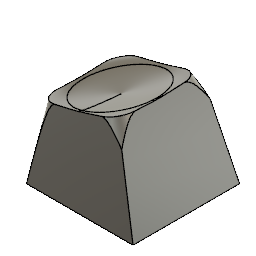
C64 Key Replacement v2 (Autodesk Fusion 360 design; units mm, degrees)
Autodesk Fusion 360 part; units mm, degrees
sketch "Sketch1" plane through (0, 0, 0) normal (0, 1, 0) x (1, 0, 0)
  line L0 (0, 0) -> (18, 0)
  line L1 (18, 0) -> (18, 18)
  line L2 (18, 18) -> (0, 18)
  line L3 (0, 18) -> (0, 0)
  dimension "d1" = 18
  dimension "d2" = 18
  constraint horizontal L0
  constraint vertical L1
  constraint horizontal L2
  constraint vertical L3
  constraint coincident L0.start L3.end
  measures "d1" distance of L0.start L0.end
  measures "d2" distance of L0.start L2.end
extrude "Extrude1" add sketch "Sketch1" along normal blind 15 contours L0 L1 L2 L3 picked at (6, 12)
sketch "Sketch2" plane through (0, 0, 0) normal (0, 0, 1) x (1, 0, 0)
  line L0 (0, 0) -> (0, 11.25)
  line L1 (0, 15) -> (18, 15)
  line L2 (18, 15) -> (0, 15)
  line L3 (0, 11.25) -> (13.507779, 15)
  line L4 (0, 0) -> (0, 6.2)
  spline S0 degree 5 poles (13.507779, 15) (13.660726, 14.651818) (13.961323, 13.959498) (14.396337, 12.933144) (14.944058, 11.589334) (15.571035, 9.953608) (16.134524, 8.366359) (16.628192, 6.832422) (17.046816, 5.355785) (17.390291, 3.936529) (17.663, 2.571306) (17.828559, 1.519298) (17.92492, 0.751524) (17.977, 0.248961) (18, 0) knots 0 0 0 0 0 0 0.1 0.2 0.3 0.4 0.5 0.6 0.7 0.8 0.9 1 1 1 1 1 1
  line L5 (18, 0) -> (0, 0)
  point P0 (16.8, 6.2)
  point P1 (18, 0)
  dimension "d5" = 11.25
  dimension "d7" = 16.8
  constraint coincident L0.start L4.start
  constraint coincident P1 S0.end
  measures "d5" distance of L0.start L0.end
  measures "d7" distance of L4.end P0
extrude "Extrude2" cut sketch "Sketch2" against normal blind 18 contours L0 L3 L4 S0 L5 picked at (9.950869, 9.63052) keep common part
move_body "Move1" bodies 1 to x (-0.96363045, 0.26723838, 0) y (-0.26723838, -0.96363045, 0) z (0, 0, 1) at (14.506577, 23.659133, 0)
move_body "Move2" bodies 1 to x (1, 0, 0) y (0, 1, 0) z (0, 0, 1) at (0, -13, 0)
sketch "Sketch3" plane through (0, 0, 0) normal (1, 0, 0) x (0, 0, -1)
  line L0 (18, -0.181709) -> (0, -0.181709)
  line L1 (9, -0.181709) -> (15.999997, -0.187866)
  line L2 (9, -0.181709) -> (2.000003, -0.18822)
  line L3 (0, 15.469424) -> (18, 15.469424)
  line L4 (0, 15.469424) -> (0, 10.659133)
  line L5 (2.000003, -0.18822) -> (0, 10.659133)
  line L6 (0, 10.659133) -> (0, 15.469424)
  line L7 (15.999997, -0.187866) -> (18, 10.659133)
  line L8 (18, 10.659133) -> (18, 15.469424)
  point P0 (0, 10.659133)
  point P1 (0, 10.659133)
  point P2 (18, 10.659133)
  dimension "d10" = 7
  dimension "d11" = 7
extrude "Extrude3" cut sketch "Sketch3" along normal mid plane 130 contours L0 L3 L4 L5 L6 L7 L8 picked at (9, 7.045519) keep common part
loft "Loft1" cut section 1 face at (6.827078, -0.181709, -11.333689) section 2 face at (8.724795, 12.262564, -12) keep common part
sketch "Sketch4" plane through (0, -0.181709, 0) normal (0, -1, 0) x (1, 0, 0)
  line L0 (11.500146, -16.001132) -> (11.500146, -1.998803)
  line L1 (11.500146, -1.998803) -> (-2.519057, -1.998803)
  line L2 (-2.519057, -16.001132) -> (11.500146, -16.001132)
  line L3 (0.480943, -1.998803) -> (8.500146, -1.998803)
  line L4 (11.500146, -4.998803) -> (11.500146, -13.001132)
  line L5 (8.500146, -16.001132) -> (0.480943, -16.001132)
  line L6 (-2.519057, -13.001132) -> (-2.519057, -4.998803)
  arc A0 (0.480943, -1.998803) -> (-2.519057, -4.998803) centre (0.480943, -4.998803) ccw
  arc A1 (11.500146, -4.998803) -> (8.500146, -1.998803) centre (8.500146, -4.998803) ccw
  arc A2 (-2.519057, -13.001132) -> (0.480943, -16.001132) centre (0.480943, -13.001132) ccw
  arc A3 (8.500146, -16.001132) -> (11.500146, -13.001132) centre (8.500146, -13.001132) ccw
  dimension "d17" = 3
  dimension "d18" = 3
  dimension "d19" = 3
  dimension "d20" = 3
  constraint horizontal L3
  constraint vertical L4
  constraint horizontal L5
  constraint vertical L6
  constraint tangent L3 A0
  constraint tangent L6 A0
  constraint tangent L3 A1
  constraint tangent L4 A1
  constraint tangent L5 A2
  constraint tangent L6 A2
  constraint tangent L4 A3
  constraint tangent L5 A3
  measures "d17" radius of A0
  measures "d18" radius of A1
  measures "d19" radius of A2
  measures "d20" radius of A3
extrude "Extrude5" cut sketch "Sketch4" against normal blind 18 draft 24 contours L0 L1 L2 L3 L4 L5 L6 A0 A1 A2 A3 picked at (5.827078, -6.666246) keep common part
move_body "Move3" bodies 1 to x (1, 0, 0) y (0, 1, 0) z (0, 0, 1) at (-5, 0, 9)
move_body "Move4" bodies 1 to x (1, 0, 0) y (0, 1, 0) z (0, 0, 1) at (0.5, 0, 0)
sketch "Sketch12" plane through (0, 0, 0) normal (1, 0, 0) x (0, 0, -1)
  line L0 (4.001132, -0.181709) -> (-4.001197, -0.181709)
  line L1 (-0.000032, -0.181709) -> (-7.000032, -0.181709)
  line L2 (-0.000032, -0.181709) -> (-0.000032, 0.818291)
  line L3 (-0.000032, -0.181709) -> (-0.000032, -1.181709)
  spline S0 degree 5 poles (-0.000032, 0.818291) (-0.530966, 0.778291) (-1.546466, 0.698291) (-2.930622, 0.578291) (-4.493362, 0.418291) (-5.943462, 0.218291) (-6.845255, 0.018291) (-7.153995, -0.181709) (-6.845255, -0.381709) (-5.943462, -0.581709) (-4.493362, -0.781709) (-2.930622, -0.941709) (-1.546466, -1.061709) (-0.530966, -1.141709) (-0.000032, -1.181709) knots 0 0 0 0 0 0 0.1 0.2 0.3 0.4 0.5 0.6 0.7 0.8 0.9 1 1 1 1 1 1
  dimension "d39" = 7
  dimension "d40" = 1
  dimension "d41" = 1
revolve "Revolve1" cut sketch "Sketch12" angle 360 about axis through (0, 1.75, 0) along (0, 1, 0) contours L0 L1 L3 S0 | L0 L1 L2 S0 picked at (-1.333754, -0.515043) picked at (-1.333754, 0.151624)
fillet "Fillet1" radius 9 1 edges at (0.002869, -0.181709, -7.000032)
move_body "Move5" bodies 1 to x (-0.96363045, -0.26723838, 0) y (0.26723838, -0.96363045, 0) z (0, 0, 1) at (-16.987899, -2.690714, 0)
move_body "Move6" bodies 1 to x (1, 0, 0) y (0, 1, 0) z (0, 0, 1) at (0, 16, 0)
move_body "Move7" bodies 1 to x (1, 0, 0) y (0, 1, 0) z (0, 0, 1) at (14, 0, 0)
sketch "Sketch13" plane through (0, 0, 0) normal (0, 1, 0) x (1, 0, 0)
  line L0 (8.217987, -9) -> (8.217987, 9)
  line L1 (-9.782013, -9) -> (8.217987, -9)
  line L2 (-9.782013, 9) -> (-9.782013, -9)
  line L3 (8.217987, 9) -> (-9.782013, 9)
  line L4 (6.317987, -7.1) -> (-7.882013, -7.1)
  line L5 (-7.882013, -7.1) -> (-7.882013, 7.1)
  line L6 (-7.882013, 7.1) -> (6.317987, 7.1)
  line L7 (6.317987, 7.1) -> (6.317987, -7.1)
  line L8 (6.317987, -7.1) -> (-7.882013, 7.1) construction
  line L9 (-7.882013, -7.1) -> (6.317987, 7.1) construction
  point P0 (-0.782013, 0)
  constraint perpendicular L4 L5
  constraint parallel L4 L6
  constraint parallel L5 L7
  constraint horizontal L4
extrude "Extrude6" cut sketch "Sketch13" along normal blind 5.5 contours L4 L5 L6 L7 picked at (-3.148679, 2.366667)
sketch "Sketch14" plane through (0, 0, 0) normal (0, 1, 0) x (1, 0, 0)
  line L0 (-7.882013, 7.1) -> (-7.882013, -7.1)
  line L1 (6.317987, -7.1) -> (6.317987, 7.1)
  line L2 (6.317987, 7.1) -> (-7.882013, 7.1)
  circle A0 centre (-0.782013, 0) radius 3.15
  dimension "d50" = 6.3
  measures "d50" diameter of A0
extrude "Extrude7" cut sketch "Sketch14" along normal blind 9 contours A0 picked at (-0.860479, 0.907771)
